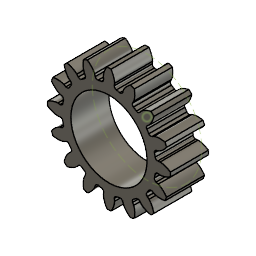
16 T (Autodesk Fusion 360 design; units mm, degrees)
description: Spur Gear; Module: 1.4375000000000002; Num Teeth: 16; Pressure Angle: 20.0; Backlash: 0.15 mm
part number: 2026-07-18-12-11-54-694
Autodesk Fusion 360 part; units mm, degrees
sketch "Base Circle" plane through (0, 0, 0) normal (0, 0, 1) x (1, 0, 0)
  circle A0 centre (0, 0) radius 9.8368
  circle A1 centre (0, 0) radius 8
extrude "Extrude1" add sketch "Base Circle" along normal blind 8
sketch "Gear Tooth" plane through (0, 0, 0) normal (0, 0, 1) x (1, 0, 0)
  spline S0 degree 5 poles (10.7414, -1.1844) (10.7476, -1.185) (10.7601, -1.1862) (10.7788, -1.1875) (10.8038, -1.1882) (10.8351, -1.1876) (10.8665, -1.186) (10.898, -1.1838) (10.9294, -1.1813) (10.9609, -1.1785) (10.9924, -1.1755) (11.024, -1.1722) (11.0555, -1.1684) (11.0871, -1.1642) (11.1187, -1.1595) (11.1503, -1.1543) (11.1819, -1.1487) (11.2135, -1.1428) (11.2451, -1.1366) (11.2768, -1.1301) (11.3084, -1.1234) (11.34, -1.1164) (11.3716, -1.109) (11.4032, -1.1014) (11.4348, -1.0934) (11.4665, -1.0852) (11.4981, -1.0767) (11.5297, -1.0679) (11.5612, -1.0588) (11.5928, -1.0495) (11.6244, -1.0399) (11.656, -1.0301) (11.6875, -1.02) (11.719, -1.0097) (11.7505, -0.9992) (11.7821, -0.9883) (11.8135, -0.9773) (11.845, -0.966) (11.8765, -0.9545) (11.9079, -0.9427) (11.9393, -0.9307) (11.9707, -0.9185) (12.0021, -0.9061) (12.0335, -0.8934) (12.0648, -0.8805) (12.0961, -0.8674) (12.1274, -0.8541) (12.1586, -0.8406) (12.1899, -0.8268) (12.2211, -0.8128) (12.2523, -0.7987) (12.2834, -0.7843) (12.3146, -0.7697) (12.3457, -0.7549) (12.3767, -0.7399) (12.4078, -0.7247) (12.4388, -0.7093) (12.4697, -0.6937) (12.5007, -0.6779) (12.5316, -0.6619) (12.5625, -0.6457) (12.5933, -0.6293) (12.6241, -0.6127) (12.6549, -0.5959) (12.6856, -0.5789) (12.7163, -0.5617) (12.747, -0.5444) (12.7776, -0.5268) (12.8082, -0.5091) (12.8388, -0.4911) (12.8693, -0.473) (12.8936, -0.4584) (12.9119, -0.4473) (12.9241, -0.4399) (12.9301, -0.4362) knots 0 0 0 0 0 0 0.01428571 0.02857143 0.04285714 0.05714286 0.07142857 0.08571429 0.1 0.11428571 0.12857143 0.14285714 0.15714286 0.17142857 0.18571429 0.2 0.21428571 0.22857143 0.24285714 0.25714286 0.27142857 0.28571429 0.3 0.31428571 0.32857143 0.34285714 0.35714286 0.37142857 0.38571429 0.4 0.41428571 0.42857143 0.44285714 0.45714286 0.47142857 0.48571429 0.5 0.51428571 0.52857143 0.54285714 0.55714286 0.57142857 0.58571429 0.6 0.61428571 0.62857143 0.64285714 0.65714286 0.67142857 0.68571429 0.7 0.71428571 0.72857143 0.74285714 0.75714286 0.77142857 0.78571429 0.8 0.81428571 0.82857143 0.84285714 0.85714286 0.87142857 0.88571429 0.9 0.91428571 0.92857143 0.94285714 0.95714286 0.97142857 0.98571429 1 1 1 1 1 1
  spline S1 degree 5 poles (10.7414, 1.1844) (10.7476, 1.185) (10.7601, 1.1862) (10.7788, 1.1875) (10.8038, 1.1882) (10.8351, 1.1876) (10.8665, 1.186) (10.898, 1.1838) (10.9294, 1.1813) (10.9609, 1.1785) (10.9924, 1.1755) (11.024, 1.1722) (11.0555, 1.1684) (11.0871, 1.1642) (11.1187, 1.1595) (11.1503, 1.1543) (11.1819, 1.1487) (11.2135, 1.1428) (11.2451, 1.1366) (11.2768, 1.1301) (11.3084, 1.1234) (11.34, 1.1164) (11.3716, 1.109) (11.4032, 1.1014) (11.4348, 1.0934) (11.4665, 1.0852) (11.4981, 1.0767) (11.5297, 1.0679) (11.5612, 1.0588) (11.5928, 1.0495) (11.6244, 1.0399) (11.656, 1.0301) (11.6875, 1.02) (11.719, 1.0097) (11.7505, 0.9992) (11.7821, 0.9883) (11.8135, 0.9773) (11.845, 0.966) (11.8765, 0.9545) (11.9079, 0.9427) (11.9393, 0.9307) (11.9707, 0.9185) (12.0021, 0.9061) (12.0335, 0.8934) (12.0648, 0.8805) (12.0961, 0.8674) (12.1274, 0.8541) (12.1586, 0.8406) (12.1899, 0.8268) (12.2211, 0.8128) (12.2523, 0.7987) (12.2834, 0.7843) (12.3146, 0.7697) (12.3457, 0.7549) (12.3767, 0.7399) (12.4078, 0.7247) (12.4388, 0.7093) (12.4697, 0.6937) (12.5007, 0.6779) (12.5316, 0.6619) (12.5625, 0.6457) (12.5933, 0.6293) (12.6241, 0.6127) (12.6549, 0.5959) (12.6856, 0.5789) (12.7163, 0.5617) (12.747, 0.5444) (12.7776, 0.5268) (12.8082, 0.5091) (12.8388, 0.4911) (12.8693, 0.473) (12.8936, 0.4584) (12.9119, 0.4473) (12.9241, 0.4399) (12.9301, 0.4362) knots 0 0 0 0 0 0 0.01428571 0.02857143 0.04285714 0.05714286 0.07142857 0.08571429 0.1 0.11428571 0.12857143 0.14285714 0.15714286 0.17142857 0.18571429 0.2 0.21428571 0.22857143 0.24285714 0.25714286 0.27142857 0.28571429 0.3 0.31428571 0.32857143 0.34285714 0.35714286 0.37142857 0.38571429 0.4 0.41428571 0.42857143 0.44285714 0.45714286 0.47142857 0.48571429 0.5 0.51428571 0.52857143 0.54285714 0.55714286 0.57142857 0.58571429 0.6 0.61428571 0.62857143 0.64285714 0.65714286 0.67142857 0.68571429 0.7 0.71428571 0.72857143 0.74285714 0.75714286 0.77142857 0.78571429 0.8 0.81428571 0.82857143 0.84285714 0.85714286 0.87142857 0.88571429 0.9 0.91428571 0.92857143 0.94285714 0.95714286 0.97142857 0.98571429 1 1 1 1 1 1
  arc A0 (12.9301, -0.4362) -> (12.9301, 0.4362) centre (0, 0) ccw
  line L0 (9.7676, -1.077) -> (10.7414, -1.1844)
  line L1 (9.7676, 1.077) -> (10.7414, 1.1844)
  line L2 (9.7676, -1.077) -> (9.7676, 1.077)
  point P0 (10.8945, -1.184)
  point P1 (11.0492, -1.1691)
  point P2 (11.2048, -1.1444)
  point P3 (11.3611, -1.1114)
  point P4 (11.5179, -1.0711)
  point P5 (11.6749, -1.024)
  point P6 (11.8322, -0.9705)
  point P7 (11.9896, -0.911)
  point P8 (12.147, -0.8456)
  point P9 (12.3043, -0.7745)
  point P10 (12.4613, -0.6979)
  point P11 (12.618, -0.6159)
  point P12 (12.7743, -0.5286)
  point P13 (10.8945, 1.184)
  point P14 (11.0492, 1.1691)
  point P15 (11.2048, 1.1444)
  point P16 (11.3611, 1.1114)
  point P17 (11.5179, 1.0711)
  point P18 (11.6749, 1.024)
  point P19 (11.8322, 0.9705)
  point P20 (11.9896, 0.911)
  point P21 (12.147, 0.8456)
  point P22 (12.3043, 0.7745)
  point P23 (12.4613, 0.6979)
  point P24 (12.618, 0.6159)
  point P25 (12.7743, 0.5286)
extrude "Extrude2" add sketch "Gear Tooth" along normal blind 8
fillet "Fillet1" radius 0.5 2 edges at (9.7776, -1.0781, 4) (9.7776, 1.0781, 4)
pattern_circular "C-Pattern1" count 16 over 360 about axis through (0, 0, 0) along (0, 0, 1) of "Extrude2", "Fillet1"
sketch "Diametrial Pitch Circle" plane through (0, 0, 0) normal (0, 0, 1) x (1, 0, 0)
  circle A0 centre (0, 0) radius 11.5 construction
named bodies: "Spur Gear (16 teeth)"
